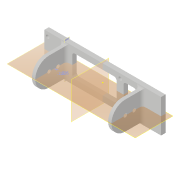
# Autodesk Inventor part: phone mount pivot
Saved by Autodesk Inventor 2018 (Build 220112000, 112)
## iProperties
Created: 2019-02-12
Part Number: phone mount pivot
Material: Generic
Document SubType Name: Modeling
Designer: ball
Density: 1 g/cm^3
Appearance: Default
Author: ball
Autodesk Inventor part; units mm, degrees
ref_plane "YZ Plane" through (0, 0, 0) normal (1, 0, 0) x (0, 1, 0)
ref_plane "XZ Plane" through (0, 0, 0) normal (0, 1, 0) x (-1, 0, 0)
ref_plane "Work Plane1" through (0, 0, 0) normal (0, 0, 1) x (1, 0, 0)
sketch "Sketch1" plane through (0, 0, 0) normal (0, 0, 1) x (1, 0, 0)
  line L0 (-66.675, -19.05) -> (66.675, -19.05) projected
  line L1 (66.675, -19.05) -> (66.675, 19.05) projected
  line L2 (66.675, 19.05) -> (-66.675, 19.05) projected
  line L3 (-66.675, 19.05) -> (-66.675, -19.05) projected
  circle A0 centre (61.0954, -13.4704) radius 1.778 construction
  circle A1 centre (59.7602, -6.9148) radius 1.778 construction
  circle A2 centre (57.15, 0) radius 2.032 construction
  circle A3 centre (54.5398, -6.9148) radius 1.778 construction
  circle A4 centre (53.2046, -13.4704) radius 1.778 construction
  circle A5 centre (54.5398, 6.9148) radius 1.778 construction
  circle A6 centre (53.2046, 13.4704) radius 1.778 construction
  circle A7 centre (59.7602, 6.9148) radius 1.778 construction
  circle A8 centre (61.0954, 13.4704) radius 1.778 construction
  circle A9 centre (47.625, 9.779) radius 1.778 construction
  circle A10 centre (47.625, -9.779) radius 1.778 construction
  circle A11 centre (34.1546, -13.4704) radius 1.778 construction
  circle A12 centre (42.0454, -13.4704) radius 1.778 construction
  circle A13 centre (40.7102, -6.9148) radius 1.778 construction
  circle A14 centre (38.1, 0) radius 2.032 construction
  circle A15 centre (40.7102, 6.9148) radius 1.778 construction
  circle A16 centre (42.0454, 13.4704) radius 1.778 construction
  circle A17 centre (35.4898, 6.9148) radius 1.778 construction
  circle A18 centre (34.1546, 13.4704) radius 1.778 construction
  circle A19 centre (35.4898, -6.9148) radius 1.778 construction
  circle A20 centre (34.1546, -13.4704) radius 1.778 construction
  circle A21 centre (28.575, -9.779) radius 1.778 construction
  circle A22 centre (28.575, 9.779) radius 1.778 construction
  circle A23 centre (21.6602, 6.9148) radius 1.778 construction
  circle A24 centre (16.4398, 6.9148) radius 1.778 construction
  circle A25 centre (15.1046, 13.4704) radius 1.778 construction
  circle A26 centre (22.9954, 13.4704) radius 1.778 construction
  circle A27 centre (19.05, 0) radius 2.032 construction
  circle A28 centre (21.6602, -6.9148) radius 1.778 construction
  circle A29 centre (22.9954, -13.4704) radius 1.778 construction
  circle A30 centre (15.1046, -13.4704) radius 1.778 construction
  circle A31 centre (16.4398, -6.9148) radius 1.778 construction
  circle A32 centre (9.525, -9.779) radius 1.778 construction
  circle A33 centre (9.525, 9.779) radius 1.778 construction
  circle A34 centre (3.9454, 13.4704) radius 1.778 construction
  circle A35 centre (2.6102, 6.9148) radius 1.778 construction
  circle A36 centre (-2.6102, 6.9148) radius 1.778 construction
  circle A37 centre (-3.9454, 13.4704) radius 1.778 construction
  circle A38 centre (0, 0) radius 2.032 construction
  circle A39 centre (-2.6102, -6.9148) radius 1.778 construction
  circle A40 centre (2.6102, -6.9148) radius 1.778 construction
  circle A41 centre (3.9454, -13.4704) radius 1.778 construction
  circle A42 centre (-3.9454, -13.4704) radius 1.778 construction
  circle A43 centre (-9.525, -9.779) radius 1.778 construction
  circle A44 centre (-9.525, 9.779) radius 1.778 construction
  circle A45 centre (-15.1046, 13.4704) radius 1.778 construction
  circle A46 centre (-22.9954, 13.4704) radius 1.778 construction
  circle A47 centre (-21.6602, 6.9148) radius 1.778 construction
  circle A48 centre (-16.4398, 6.9148) radius 1.778 construction
  circle A49 centre (-19.05, 0) radius 2.032 construction
  circle A50 centre (-21.6602, -6.9148) radius 1.778 construction
  circle A51 centre (-16.4398, -6.9148) radius 1.778 construction
  circle A52 centre (-15.1046, -13.4704) radius 1.778 construction
  circle A53 centre (-22.9954, -13.4704) radius 1.778 construction
  circle A54 centre (-28.575, -9.779) radius 1.778 construction
  circle A55 centre (-28.575, 9.779) radius 1.778 construction
  circle A56 centre (-34.1546, 13.4704) radius 1.778 construction
  circle A57 centre (-42.0454, 13.4704) radius 1.778 construction
  circle A58 centre (-40.7102, 6.9148) radius 1.778 construction
  circle A59 centre (-35.4898, 6.9148) radius 1.778 construction
  circle A60 centre (-38.1, 0) radius 2.032 construction
  circle A61 centre (-35.4898, -6.9148) radius 1.778 construction
  circle A62 centre (-40.7102, -6.9148) radius 1.778 construction
  circle A63 centre (-34.1546, -13.4704) radius 1.778 construction
  circle A64 centre (-42.0454, -13.4704) radius 1.778 construction
  circle A65 centre (-47.625, -9.779) radius 1.778 construction
  circle A66 centre (-53.2046, -13.4704) radius 1.778 construction
  circle A67 centre (-54.5398, -6.9148) radius 1.778 construction
  circle A68 centre (-57.15, 0) radius 2.032 construction
  circle A69 centre (-59.7602, -6.9148) radius 1.778 construction
  circle A70 centre (-61.0954, -13.4704) radius 1.778 construction
  circle A71 centre (-59.7602, 6.9148) radius 1.778 construction
  circle A72 centre (-54.5398, 6.9148) radius 1.778 construction
  circle A73 centre (-53.2046, 13.4704) radius 1.778 construction
  circle A74 centre (-61.0954, 13.4704) radius 1.778 construction
extrude "Extrusion2" add sketch "Sketch1" along normal blind 5.08
sketch "Sketch2" plane through (0, 0, 5.08) normal (0, 0, 1) x (1, 0, 0)
  circle A0 centre (-53.2046, -13.4704) radius 1.9685 construction
  circle A1 centre (-53.2046, -13.4704) radius 2.8702 construction
  circle A2 centre (-42.0454, -13.4704) radius 1.9685 construction
  circle A3 centre (-42.0454, -13.4704) radius 2.8702 construction
  point P0 (0, 0)
  dimension "d37" = 5.7404
  dimension "d38" = 5.7404
  constraints: 2 centre point, 2 coincident
  measures "d37" diameter of A1
  measures "d38" diameter of A3
ref_plane "Work Plane2" through (-43.561, -19.05, 0) normal (-1, 0, 0) x (0, 0, 1)
sketch "Sketch3" plane through (-43.561, -19.05, 0) normal (-1, 0, 0) x (0, 0, 1)
  line L0 (0, 6.35) -> (5.08, 6.35) construction
  line L1 (5.08, 0) -> (5.08, 38.1) projected
  line L2 (0, 0) -> (5.08, 0) projected
  line L3 (0, 0) -> (0, 38.1) projected
  line L4 (0, 31.75) -> (5.08, 31.75) construction
  line L5 (0, 38.1) -> (5.08, 38.1) projected
  line L6 (8.89, 31.75) -> (8.89, 6.35) construction
  circle A0 centre (24.765, 19.05) radius 15.875
  circle A1 centre (24.765, 19.05) radius 1.9685
  line L7 (24.765, 19.05) -> (34.925, 19.05) construction
  line L8 (24.765, 34.925) -> (5.08, 34.925)
  line L9 (5.08, 34.925) -> (5.08, 3.175)
  line L10 (5.08, 3.175) -> (23.495, 3.175)
  arc A2 (24.765, 31.75) -> (23.495, 6.4137) centre (24.765, 19.05) ccw
  line L11 (24.765, 31.75) -> (24.765, 34.925)
  line L12 (23.495, 3.175) -> (23.495, 6.4137)
  line L13 (24.765, 17.0815) -> (24.765, 21.0185)
  line L14 (5.08, 21.0185) -> (5.08, 17.0815) projected
  line L15 (5.08, 19.05) -> (5.08, 29.21)
  line L16 (5.08, 19.05) -> (5.08, 8.89)
  circle A3 centre (14.605, 19.05) radius 1.9685
  point P0 (0, 19.05)
  dimension "d45" = 31.75
  dimension "d40" = 6.35
  dimension "d41" = 6.35
  dimension "d43" = 15.875
  dimension "d46" = 3.937
  dimension "d51" = 3.81
  dimension "d52" = 19.05
  dimension "d61" = 25.4
  dimension "d62" = 10.16
  dimension "d63" = 10.16
  dimension "d66" = 10.16
  dimension "d67" = 3.937
  constraints: 24 end point, 6 point on line, 5 coincident, 4 parallel, 4 point on circle, 3 centre point, 3 horizontal, 2 perpendicular, 1 midpoint, 1 vertical alignment, 2 other
  measures "d40" distance between parallel lines of L2 L0
  measures "d41" distance between parallel lines of L5 L4
  measures "d43" distance from line of L6 point (24.765, 19.05)
  measures "d46" diameter of A1
  measures "d51" distance between parallel lines of L1 L6
  measures "d52" distance from line of L5 point (24.765, 19.05)
  measures "d61" diameter of A2
  measures "d62" distance of L15.start L15.end
  measures "d63" distance of L15.start L16.end
  measures "d66" distance of point (24.765, 19.05) point (14.605, 19.05)
  measures "d67" diameter of A3
ref_plane "Work Plane3" through (0, -19.05, 0) normal (1, 0, 0) x (0, 0, -1)
extrude "Extrusion4" add sketch "Sketch3" along normal blind 1.905 and the other way blind 1.905 contours L1 L8 A0 L12 L10 | L12 A2 L11 A0 | A0 L11 A2 L12
mirror "Mirror2" about plane through (0, -19.05, 0) normal (1, 0, 0) of "Extrusion4"
fillet "Fillet3" radius 3.175 8 edges at (-41.656, 0, 5.08) (-43.561, -15.875, 5.08) (-45.466, 0, 5.08) (-43.561, 15.875, 5.08) (41.656, 0, 5.08) (43.561, 15.875, 5.08) (45.466, 0, 5.08) (43.561, -15.875, 5.08)
ref_plane "Work Plane4" through (-66.675, 0, 0) normal (0, 1, 0) x (1, 0, 0)
sketch "Sketch5" plane through (0, 0, 0) normal (0, 0, -1) x (-1, 0, 0)
  line L0 (66.675, 19.05) -> (66.675, -19.05) projected
  line L1 (-66.675, 19.05) -> (66.675, 19.05) projected
  line L2 (66.675, -19.05) -> (-66.675, -19.05) projected
  point P0 (0, 0)
  point P1 (62.9666, 13.97)
  point P2 (62.9666, -13.97)
  dimension "d73" = 3.7084
  dimension "d74" = 3.7084
  dimension "d75" = 5.08
  dimension "d76" = 5.08
  measures "d73" distance from line of L0 point (62.967, 13.97)
  measures "d74" distance from line of L0 point (62.967, -13.97)
  measures "d75" distance from line of L1 point (62.967, 13.97)
  measures "d76" distance from line of L2 point (62.967, -13.97)
hole "Hole1" at (-62.9666, -13.97, 0) at (-62.9666, 13.97, 0) direction (0, 0, 1) diameter 3.937 end through all
sketch "Sketch6" plane through (0, 0, 5.08) normal (0, 0, 1) x (1, 0, 0)
  line L0 (15.875, 12.7) -> (-34.925, 12.7)
  line L1 (-34.925, 12.7) -> (-34.925, -12.7)
  line L2 (-34.925, -12.7) -> (15.875, -12.7)
  line L3 (15.875, -12.7) -> (15.875, 12.7)
  line L4 (-38.481, -19.05) -> (38.481, -19.05) projected
  line L5 (38.481, 19.05) -> (-38.481, 19.05) projected
  line L6 (-66.675, 19.05) -> (-66.675, -19.05) projected
  line L7 (66.675, -19.05) -> (66.675, 19.05) projected
  line L8 (23.7236, -12.7) -> (38.481, -12.7)
  line L9 (38.481, 12.7) -> (23.7236, 12.7)
  line L10 (23.7236, 12.7) -> (23.7236, -12.7)
  line L11 (38.481, 19.05) -> (38.481, -19.05) projected
  line L12 (38.481, -12.7) -> (38.481, 12.7)
  point P0 (0, 0)
  dimension "d84" = 6.35
  dimension "d85" = 6.35
  dimension "d86" = 31.75
  dimension "d87" = 50.8
  dimension "d102" = 42.9514
  constraints: 16 end point, 3 parallel, 2 horizontal, 1 perpendicular, 1 point on line
  measures "d84" distance between parallel lines of L4 L2
  measures "d85" distance between parallel lines of L5 L0
  measures "d86" distance between parallel lines of L6 L1
  measures "d87" distance between parallel lines of L7 L3
  measures "d102" distance between parallel lines of L7 L10
extrude "Extrusion5" cut sketch "Sketch6" against normal through all
fillet "Fillet4" radius 3.175 4 edges at (15.875, -12.7, 2.54) (-34.925, -12.7, 2.54) (-34.925, 12.7, 2.54) (15.875, 12.7, 2.54)
sketch "Sketch7" plane through (0, 0, 0) normal (0, 0, -1) x (-1, 0, 0)
  line L0 (-66.675, -19.05) -> (-66.675, 19.05) projected
  line L1 (66.675, -19.05) -> (-66.675, -19.05) projected
  line L2 (-66.675, 19.05) -> (66.675, 19.05) projected
  point P0 (0, 0)
  point P1 (-20.0406, 13.97)
  point P2 (-20.0406, -13.97)
  dimension "d91" = 46.6344
  dimension "d92" = 46.6344
  dimension "d93" = 5.08
  dimension "d94" = 5.08
  measures "d91" distance from line of L0 point (-20.041, 13.97)
  measures "d92" distance from line of L0 point (-20.041, -13.97)
  measures "d93" distance from line of L1 point (-20.041, -13.97)
  measures "d94" distance from line of L2 point (-20.041, 13.97)
hole "Hole2" at (20.0406, 13.97, 0) at (20.0406, -13.97, 0) direction (0, 0, 1) diameter 3.937 end through all
fillet "Fillet5" radius 3.175 4 edges at (38.481, 12.7, 2.54) (23.7236, 12.7, 2.54) (38.481, -12.7, 2.54) (23.7236, -12.7, 2.54)
body "Solid2"
